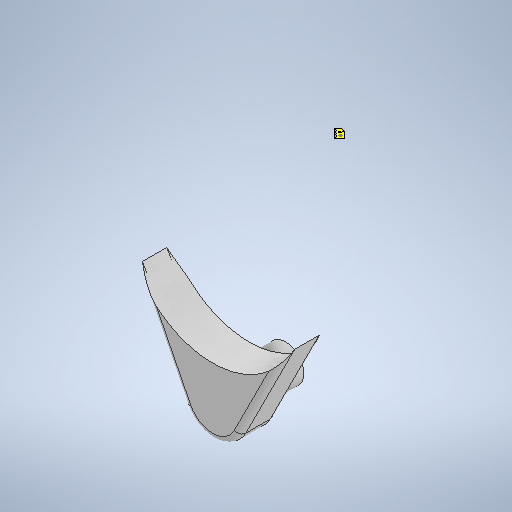
# Autodesk Inventor part: Joystick Extra Hook
Saved by Autodesk Inventor 2025.2 (Build 292293000, 293)
## iProperties
Created: 2025-03-11
Part Number: Joystick Extra Hook
Material: Generic
Document SubType Name: Modeling
Designer: eason
Density: 1 g/cm^3
Appearance: Default
Author: eason
Autodesk Inventor part; units mm, degrees
ref_plane "YZ Plane" through (0, 0, 0) normal (1, 0, 0) x (0, 1, 0)
ref_plane "XZ Plane" through (0, 0, 0) normal (0, 1, 0) x (-1, 0, 0)
ref_plane "XY Plane" through (0, 0, 0) normal (0, 0, 1) x (1, 0, 0)
sketch "Sketch1" plane through (0, 0, 0) normal (0, 0, 1) x (1, 0, 0)
  circle A0 centre (0, 0) radius 7
  circle A1 centre (0, -10) radius 1.5
  circle A2 centre (0, -10) radius 2.5
  line L0 (0, -16.4) -> (0, 10.9) projected
  line L1 (-2.2326, -11.125) -> (-6.2512, -3.15)
  line L2 (2.2326, -11.125) -> (6.2512, -3.15)
  dimension "d0" = 14
  dimension "d1" = 3
  dimension "d2" = 1
  dimension "d3" = 10
  constraints: 4 end point, 4 point on circle, 4 tangent, 3 centre point, 2 coincident, 1 point on line
  measures "d0" diameter of A0
  measures "d1" diameter of A1
  measures "d2" radial gap between concentric circles of A2 A1
  measures "d3" distance of point (0, 0) A1.centre
extrude "Extrusion1" add sketch "Sketch1" along normal blind 3 contours L2 A2 L0 A0 | L0 A2 L1 A0 | A2 L0 A1 | L0 A1 A2 | L0 A1 | A1 L0
extrude "Extrusion2" add sketch "Sketch1" against normal blind 3 contours L0 A1 | A1 L0
fillet "Fillet1" radius 0.5 6 edges at (0, -12.5, 3) (-4.2419, -7.1375, 3) (4.2419, -7.1375, 3) (0, -12.5, 0) (-4.2419, -7.1375, 0) (4.2419, -7.1375, 0)
body "Solid1"
